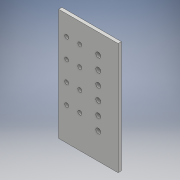
# Autodesk Inventor part: Switchboard
Saved by Autodesk Inventor 2018 (Build 220112000, 112)
## iProperties
Created: 2017-12-06
Part Number: Switchboard
Material: Generic
Document SubType Name: Modeling
Designer: a
Density: 1 g/cm^3
Appearance: Default
Author: a
Autodesk Inventor part; units mm, degrees
ref_plane "YZ Plane" through (0, 0, 0) normal (1, 0, 0) x (0, 1, 0)
ref_plane "XZ Plane" through (0, 0, 0) normal (0, 1, 0) x (-1, 0, 0)
ref_plane "XY Plane" through (0, 0, 0) normal (0, 0, 1) x (1, 0, 0)
sketch "Sketch1" plane through (0, 0, 0) normal (0, 1, 0) x (-1, 0, 0)
  line L0 (0, 0) -> (150, 0)
  line L1 (150, 0) -> (150, -170)
  line L2 (150, -170) -> (0, -170)
  line L3 (0, -170) -> (0, 0)
  dimension "d0" = 150
  dimension "d1" = 170
  constraints: 8 end point, 2 parallel, 1 horizontal, 1 perpendicular
  measures "d0" distance of L1.end L2.end
  measures "d1" distance of L0.end L1.end
extrude "Extrusion1" add sketch "Sketch1" along normal blind 5
sketch "Sketch2" plane through (0, 5, 0) normal (0, 1, 0) x (1, 0, 0)
  circle A0 centre (-30, 30) radius 3.75
  point P0 (0, 0)
  dimension "d4" = 7.5
  constraints: 1 centre point
  measures "d4" diameter of A0
extrude "Extrusion2" cut sketch "Sketch2" against normal blind 5
pattern_linear "Rectangular Pattern1" count 6 spacing 20 along (0, 0, -1) of "Extrusion2"
sketch "Sketch3" plane through (0, 5, 0) normal (0, 1, 0) x (1, 0, 0)
  circle A0 centre (-58, 30) radius 3
  point P0 (0, 0)
  dimension "d10" = 6
  constraints: 1 centre point
  measures "d10" diameter of A0
extrude "Extrusion3" cut sketch "Sketch3" against normal blind 5
pattern_linear "Rectangular Pattern2" count 2 spacing 20 along (-1, 0, 0) count 4 spacing 30 along (0, 0, -1) of "Extrusion3"
sketch "Sketch4" plane through (-150, 0, -170) normal (-1, 0, 0) x (0, 0, 1)
  line L0 (170, 5) -> (0, 5) projected
  line L1 (170, 0) -> (0, 0)
  line L2 (0, 0) -> (0, 5)
  line L3 (0, 5) -> (170, 5)
  line L4 (170, 5) -> (170, 0)
  constraints: 8 end point, 2 parallel, 1 horizontal, 1 perpendicular
extrude "Extrusion4" cut sketch "Sketch4" against normal blind 59.75
body "Solid1"
